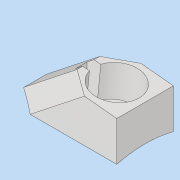
# Autodesk Inventor part: electromagnetHolder
Saved by Autodesk Inventor 2017.3 (Build 213256000, 256)
## iProperties
Created: 2018-08-28
Part Number: electromagnetHolder
Material: ABS Plastic
Document SubType Name: Modeling
Designer: Derek Wider
Density: 1.06 g/cm^3
Appearance: Smooth - White
Author: Derek Wider
Autodesk Inventor part; units mm, degrees
ref_plane "YZ Plane" through (0, 0, 0) normal (1, 0, 0) x (0, 1, 0)
ref_plane "XZ Plane" through (0, 0, 0) normal (0, 1, 0) x (-1, 0, 0)
ref_plane "XY Plane" through (0, 0, 0) normal (0, 0, 1) x (1, 0, 0)
sketch "Sketch1" plane through (0, 0, 0) normal (0, 0, 1) x (1, 0, 0)
  line L0 (0, 0) -> (0, 20.32)
  line L1 (0, 20.32) -> (25.4, 17.78)
  line L2 (25.4, 17.78) -> (25.4, 0)
  line L3 (25.4, 0) -> (0, 0)
  dimension "d0" = 20.32
  dimension "d1" = 25.4
  dimension "d2" = 17.78
  constraints: 8 end point, 1 parallel, 1 perpendicular, 1 vertical
  measures "d0" distance of L0.start L0.end
  measures "d1" distance of L2.end L0.start
  measures "d2" distance of L1.end L2.end
extrude "Extrusion1" add sketch "Sketch1" along normal blind 25.4
sketch "Sketch2" plane through (0, 0, 0) normal (-1, 0, 0) x (0, 0, 1)
  line L0 (0, 0) -> (25.4, 0) construction
  arc A0 (25.4, 0) -> (0, 0) centre (12.7, -49.1869) ccw
  line L1 (0, 0) -> (25.4, 0)
  point P0 (12.7, 0)
  dimension "d5" = 101.6
  constraints: 2 end point, 2 point on circle, 1 centre point, 1 horizontal, 1 midpoint, 1 vertical alignment
  measures "d5" diameter of A0
extrude "Extrusion2" cut sketch "Sketch2" against normal through all
sketch "Sketch3" plane through (0, 20.32, 25.4) normal (0.0995037, 0.9950372, 0) x (0.9950372, -0.0995037, 0)
  line L0 (0, 25.4) -> (25.5267, 25.4) construction
  line L1 (0, 25.4) -> (0, 0) construction
  line L2 (25.5267, 0) -> (0, 0) construction
  line L3 (25.5267, 25.4) -> (25.5267, 0) construction
  circle A0 centre (12.7633, 12.7) radius 10.0838
  point P0 (2.0219, 25.4)
  point P1 (0, 12.7)
  point P2 (12.7633, 25.4)
  dimension "d8" = 20.1676
  constraints: 2 midpoint, 1 centre point, 1 horizontal alignment, 1 vertical alignment
  measures "d8" diameter of A0
extrude "Extrusion3" cut sketch "Sketch3" against normal blind 15.0876
sketch "Sketch4" plane through (0, 20.32, 0) normal (-1, 0, 0) x (0, 0, 1)
  line L0 (0, 0) -> (25.4, 0) projected
  line L1 (10.16, 0) -> (15.24, 0)
  line L2 (15.24, 0) -> (15.24, -15.24)
  line L3 (15.24, -15.24) -> (10.16, -15.24)
  line L4 (10.16, -15.24) -> (10.16, 0)
  point P0 (0, -20.32)
  point P1 (12.7, 0)
  point P2 (12.7, 0)
  dimension "d11" = 15.24
  dimension "d12" = 5.08
  constraints: 8 end point, 2 midpoint, 2 parallel, 1 coincident, 1 horizontal, 1 perpendicular, 1 point on line
  measures "d11" distance of L3.end L1.start
  measures "d12" distance of L2.end L3.end
extrude "Extrusion4" cut sketch "Sketch4" against normal up to surface round surface about axis through (12.7, 19.05, 12.7) along (-0.0995037, -0.9950372, 0) radius 10.0838 far side no
sketch "Sketch5" plane through (11.1987, 4.0373, 12.7) normal (0.0995037, 0.9950372, 0) x (0.9950372, -0.0995037, 0)
  circle A0 centre (0, 0) radius 2.54
  point P0 (-10.7414, 12.7)
  dimension "d15" = 5.08
  constraints: 1 centre point
  measures "d15" diameter of A0
extrude "Extrusion5" cut sketch "Sketch5" against normal up to surface round surface about axis through (0, -49.1869, 12.7) along (1, 0, 0) radius 50.8 far side no
ref_plane "Work Plane1" through (11.1987, 4.0373, 12.7) normal (0.9950372, -0.0995037, 0) x (-0.0995037, -0.9950372, 0)
sketch "Sketch6" plane through (11.1987, 4.0373, 12.7) normal (0.9950372, -0.0995037, 0) x (-0.0995037, -0.9950372, 0)
  line L0 (0, -2.54) -> (2.5001, -2.54) projected
  line L1 (0.762, -2.54) -> (1.651, -3.429)
  line L2 (1.651, -3.429) -> (3.302, -3.429)
  line L3 (3.302, -3.429) -> (3.302, -2.54)
  line L4 (3.302, -2.54) -> (0.762, -2.54)
  line L5 (-22.377, 0) -> (10.9571, 0) projected
  point P0 (5.1316, 12.7)
  dimension "d22" = 0.762
  dimension "d23" = 0.889
  dimension "d24" = 0.889
  dimension "d25" = 2.54
  constraints: 8 end point, 2 perpendicular, 1 parallel, 1 point on line
  measures "d22" distance of L1.start L0.start
  measures "d23" distance between parallel lines of L0 L2
  measures "d24" horizontal distance of L1.start L1.end
  measures "d25" distance of L3.end L1.start
revolve "Revolution1" cut sketch "Sketch6" angle 360 about axis through (11.1987, 4.0373, 12.7) along (-0.0995037, -0.9950372, 0)
sketch "Sketch7" plane through (0, 0, 0) normal (-1, 0, 0) x (0, 0, 1)
  line L0 (10.16, 5.08) -> (10.16, 20.32) projected
  line L1 (0, 20.32) -> (10.16, 20.32) projected
  line L2 (0, 0) -> (0, 20.32) projected
  arc A0 (25.4, 0) -> (0, 0) centre (12.7, -49.1869) ccw projected
  line L3 (25.4, 20.32) -> (25.4, 0) projected
  line L4 (15.24, 20.32) -> (25.4, 20.32) projected
  line L5 (15.24, 20.32) -> (15.24, 5.08) projected
  line L6 (15.24, 5.08) -> (10.16, 5.08) projected
  line L7 (15.24, 20.32) -> (10.16, 20.32)
  constraints: 2 end point, 1 horizontal
extrude "Extrusion6" add sketch "Sketch7" along normal blind 25.4
chamfer "Chamfer2" distance 20.066 distance2 25.4 1 edges at (-25.4, 20.32, 12.7) measured on face at (-25.4, 19.82, 12.7)
chamfer "Chamfer3" distance 7.62 angle 45 2 edges at (-12.7, 10.287, 25.4) (-12.7, 10.287, 0)
sketch "Sketch9" plane through (0, 0, 0) normal (0, 0, -1) x (-1, 0, 0)
  line L0 (0, 5.08) -> (-1.4957, 5.08) projected
  line L1 (0, 5.08) -> (3.175, 5.08)
  line L2 (3.175, 5.08) -> (3.175, 1.905)
  line L3 (3.175, 1.905) -> (0, 1.905)
  line L4 (0, 1.905) -> (0, 5.08)
  point P0 (0, 0)
  dimension "d39" = 3.175
  dimension "d40" = 3.175
  constraints: 8 end point, 2 parallel, 1 horizontal, 1 perpendicular
  measures "d39" distance of L2.end L3.end
  measures "d40" distance of L1.end L2.end
extrude "Extrusion8" cut sketch "Sketch9" against normal up to surface (15.24 mm away)
sketch "Sketch10" plane through (0, 0, 0) normal (1, 0, 0) x (0, 0, -1)
  line L0 (0, 5.08) -> (-15.24, 5.08) projected
  line L1 (-15.24, 1.905) -> (-15.24, 5.08) projected
  line L2 (-15.24, 5.08) -> (-10.16, 5.08)
  line L3 (-10.16, 5.08) -> (-10.16, 8.255)
  line L4 (-10.16, 8.255) -> (-15.24, 8.255)
  line L5 (-15.24, 8.255) -> (-15.24, 5.08)
  point P0 (0, 0)
  dimension "d43" = 3.175
  dimension "d44" = 5.08
  constraints: 8 end point, 2 parallel, 1 horizontal, 1 perpendicular
  measures "d43" distance of L2.end L3.end
  measures "d44" distance of L3.end L4.end
extrude "Extrusion9" cut sketch "Sketch10" against normal up to surface (3.175 mm away)
sketch "Sketch11" plane through (0, 0, 0) normal (1, 0, 0) x (0, 0, -1)
  line L0 (-15.24, 8.255) -> (-10.16, 8.255) projected
  line L1 (-10.16, 8.255) -> (-10.16, 20.32) projected
  line L2 (-15.24, 20.32) -> (-10.16, 20.32) projected
  line L3 (-15.24, 20.32) -> (-15.24, 8.255) projected
  point P0 (0, 0)
extrude "Extrusion10" cut sketch "Sketch11" against normal blind 3.175
body "Solid1"
